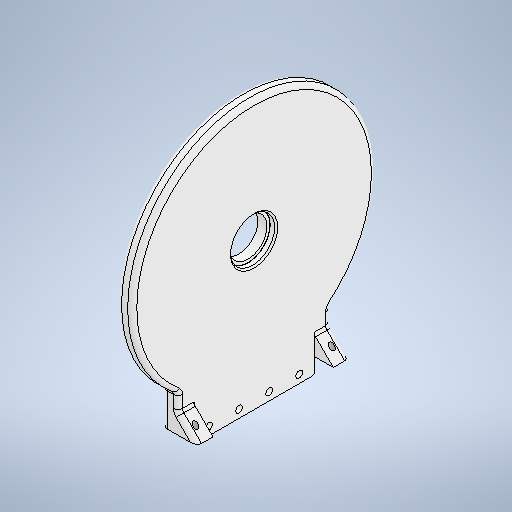
# Autodesk Inventor part: joint4_base_right
Saved by Autodesk Inventor 2025.3 (Build 293356030, 356C)
## iProperties
Created: 2025-11-08
Part Number: joint4_base_right
Material: PLA filament
Document SubType Name: Modeling
Designer: MSI
Density: 1.2 g/cm^3
Appearance: 일반
Mass: 255.844 g
Surface Area: 499.305 cm^2
Volume: 213.204 cm^3
Author: MSI
Autodesk Inventor part; units mm, degrees
ref_plane "YZ Plane" through (0, 0, 0) normal (1, 0, 0) x (0, 1, 0)
ref_plane "XZ Plane" through (0, 0, 0) normal (0, 1, 0) x (-1, 0, 0)
ref_plane "XY Plane" through (0, 0, 0) normal (0, 0, 1) x (1, 0, 0)
sketch "스케치1" plane through (0, 0, 0) normal (1, 0, 0) x (0, 1, 0)
  circle A0 centre (0, 0) radius 80
  line L0 (0, 50) -> (-96, 50)
  line L1 (-96, 50) -> (-96, -50)
  line L2 (-96, -50) -> (0, -50)
  line L3 (0, -50) -> (0, 50)
  point P0 (-62.45, -50)
  point P1 (-62.45, 50)
  dimension "d0" = 160
  dimension "d1" = 96
  dimension "d2" = 100
  constraints: 8 end point, 2 coincident, 2 parallel, 1 centre point, 1 horizontal, 1 midpoint, 1 perpendicular
  measures "d0" diameter of A0
  measures "d1" distance of L2.end L1.end
  measures "d2" distance of L1.end L0.end
extrude "돌출1" add sketch "스케치1" along normal mid plane 10
sketch "스케치2" plane through (5, 0, 0) normal (1, 0, 0) x (0, 0, -1)
  arc A0 (50, -62.45) -> (-50, -62.45) centre (0, 0) ccw projected
  constraints: 1 coincident
hole "구멍1" at (5, 0, 0) direction (-1, 0, 0) diameter 25 end through all counterbore diameter 29 counterbore depth 4
fillet "모깎기1" radius 0.1 1 edges at (1, 0, 14.5)
sketch "스케치3" plane through (-5, -96, 50) normal (0, 0, 1) x (1, 0, 0)
  line L0 (0, 0) -> (10, 0) projected
  line L1 (10, 0) -> (10, 33.55) projected
  line L2 (0, 0) -> (10, 0)
  line L3 (10, 0) -> (10, 10.5)
  line L4 (10, 10.5) -> (0, 10.5)
  line L5 (0, 10.5) -> (0, 0)
  point P0 (5, 96)
  dimension "d12" = 10.5
  constraints: 8 end point, 2 parallel, 1 horizontal, 1 perpendicular, 1 point on line
  measures "d12" distance between parallel lines of L0 L4
extrude "돌출2" cut sketch "스케치3" against normal blind 10.5
sketch "스케치5" plane through (-5, -62.45, 50) normal (0, 0, 1) x (1, 0, 0)
  line L0 (10, 0) -> (10, -23.05) projected
  line L1 (10, -10.55) -> (22.5, -23.05)
  line L2 (22.5, -23.05) -> (10, -23.05)
  point P0 (5, 62.45)
  dimension "d27" = 45
  dimension "d30" = 12.5
  constraints: 4 end point, 1 horizontal, 1 point on line
  measures "d27" angle of L2 L1
  measures "d30" distance from line of L2 L1.start
extrude "돌출3" add sketch "스케치5" against normal blind 10.5
mirror "미러1" about plane through (0, 0, 0) normal (0, 0, 1) of "돌출2", "돌출3"
sketch "스케치6" plane through (-5, -85.5, 39.5) normal (0, -1, 0) x (1, 0, 0)
  line L0 (5, 5.25) -> (16.25, 5.25)
  line L1 (16.25, 5.25) -> (16.25, -84.25)
  line L2 (16.25, -84.25) -> (5, -84.25)
  line L3 (5, -84.25) -> (5, 5.25)
  line L4 (0, 10.5) -> (10, 10.5) projected
  line L5 (22.5, 10.5) -> (10, 10.5) projected
  line L6 (22.5, -89.5) -> (10, -89.5) projected
  line L7 (10, -79) -> (10, -89.5) projected
  line L8 (10, -79) -> (22.5, -79) projected
  line L9 (22.5, -89.5) -> (22.5, -79) projected
  line L10 (22.5, 10.5) -> (10, 10.5) projected
  line L11 (22.5, 10.5) -> (22.5, 0) projected
  line L12 (10, 0) -> (22.5, 0) projected
  line L13 (10, 10.5) -> (10, 0) projected
  point P0 (5, -39.5)
  point P1 (5, 10.5)
  point P2 (16.25, 10.5)
  point P3 (22.5, 5.25)
  point P4 (22.5, -84.25)
  constraints: 8 end point, 4 coincident, 4 midpoint, 4 point on line, 2 parallel, 1 horizontal, 1 perpendicular
hole "구멍3" at (11.25, -85.5, -44.75) at (0, -85.5, -44.75) at (0, -85.5, 44.75) at (11.25, -85.5, 44.75) direction (0, 1, 0) diameter 3.242 depth 10 tip angle 118 thread size "M4x0.7" class "6H" standard "ISO Metric profile"
sketch "스케치4" plane through (-5, 0, 0) normal (-1, 0, 0) x (0, 0, 1)
  line L0 (-29.625, -90.75) -> (29.625, -90.75)
  line L1 (-39.5, -96) -> (39.5, -96) projected
  line L2 (-39.5, -85.5) -> (-39.5, -96) projected
  point P0 (0, 0)
  point P1 (0, -90.75)
  point P2 (0, -96)
  point P3 (-39.5, -90.75)
  point P4 (-9.875, -90.75)
  point P5 (9.875, -90.75)
  dimension "d17" = 59.25
  dimension "d18" = 19.75
  dimension "d19" = 19.75
  constraints: 3 midpoint, 3 point on line, 2 coincident, 2 end point, 1 horizontal, 1 vertical alignment
  measures "d17" distance of L0.start L0.end
  measures "d18" distance of point (-9.875, -90.75) point (-29.625, -90.75)
  measures "d19" distance of point (9.875, -90.75) point (29.625, -90.75)
hole "구멍2" at (-5, -90.75, -29.625) at (-5, -90.75, -9.875) at (-5, -90.75, 9.875) at (-5, -90.75, 29.625) direction (1, 0, 0) diameter 4.5 end through all counterbore diameter 8 counterbore depth 4.4 clearance for "Socket Head Cap Screw ISO 4762" size "M4" standard "ISO"
fillet "모깎기2" radius 3 4 edges at (0, -62.45, 50) (0, -62.45, -50) (5, -73, 44.75) (5, -73, -44.75)
fillet "모깎기3" radius 3 10 edges at (-5, -62.5995, -50.2846) (-5, -74.6874, -50) (-5, -62.5995, 50.2846) (-5, -74.6874, 50) (-5, 80, 0) (5, -62.5995, 50.2846) (5, -67.8161, 50) (5, -62.5995, -50.2846) (5, -67.8161, -50) (5, 80, 0)
chamfer "모따기1" distance 1 angle 45 3 edges at (0, -96, 39.5) (0, -96, -39.5) (5, 0, 14.5)
equation "\"d17\" = 3 * d18"
equation "\"d19\" = d18"
